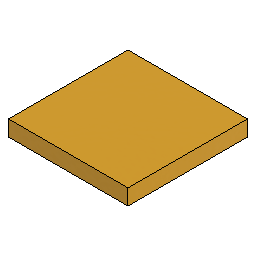
USB Container (Autodesk Fusion 360 archive; units mm, degrees)
design "Sticky Notes"
Autodesk Fusion 360 part; units mm, degrees
sketch "Sketch1" plane through (0, 0, 0) normal (0, 0, 1) x (1, 0, 0)
  line L0 (38, 38) -> (-38, 38)
  line L1 (-38, 38) -> (-38, -38)
  line L2 (-38, -38) -> (38, -38)
  line L3 (38, -38) -> (38, 38)
  line L4 (38, 38) -> (-38, -38) construction
  line L5 (-38, 38) -> (38, -38) construction
  dimension "d1" = 76
  dimension "d2" = 76
  constraint horizontal L0
  constraint perpendicular L0 L1
  constraint parallel L0 L2
  constraint parallel L1 L3
  constraint coincident L4 origin
  constraint coincident L5 origin
  measures "d1" distance of L1.end L2.end
  measures "d2" distance of L0.end L1.end
extrude "Extrude1" add sketch "Sketch1" along normal blind 10
